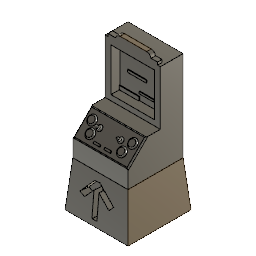
DiegoCabinet (Autodesk Fusion 360 design; units mm, degrees)
Autodesk Fusion 360 part; units mm, degrees
sketch "Sketch1" plane through (0, 0, 0) normal (0, 0, 1) x (1, 0, 0)
  line L0 (0, 50) -> (70, 50)
  line L1 (70, 50) -> (70, -20)
  line L2 (70, -20) -> (0, -20)
  line L3 (0, -20) -> (0, 50)
  constraint horizontal L0
  constraint vertical L1
  constraint horizontal L2
  constraint vertical L3
extrude "Extrude1" add sketch "Sketch1" along normal blind 50 draft -5
sketch "Sketch2" plane through (0, 0, 50) normal (0, 0, 1) x (-1, 0, 0)
  line L0 (-4.3744, -45.6256) -> (-4.3744, 15.6256)
  line L1 (-4.3744, 15.6256) -> (-65.6256, 15.6256)
  line L2 (-65.6256, 15.6256) -> (-65.6256, -45.6256)
  line L3 (-65.6256, -45.6256) -> (-4.3744, -45.6256)
  line L4 (-4.3744, 15.6256) -> (-65.6256, 15.6256)
  line L5 (-65.6256, 15.6256) -> (-65.6256, -45.6256)
  line L6 (-65.6256, -45.6256) -> (-4.3744, -45.6256)
  line L7 (-4.3744, -45.6256) -> (-4.3744, 15.6256)
  constraint horizontal L4
  constraint vertical L5
  constraint horizontal L6
  constraint vertical L7
  constraint coincident L2.end L3.start
  constraint coincident L0.end L1.start
extrude "Extrude2" add sketch "Sketch2" along normal blind 40
chamfer "Chamfer1" distance 20 angle 45 1 edges at (35, -15.6256, 90)
sketch "Sketch3" plane through (0, 0, 90) normal (0, 0, 1) x (-1, 0, 0)
  line L0 (-4.3744, -4.3744) -> (-65.6256, -4.3744)
  line L1 (-65.6256, -4.3744) -> (-65.6256, -45.6256)
  line L2 (-65.6256, -45.6256) -> (-4.3744, -45.6256)
  line L3 (-4.3744, -45.6256) -> (-4.3744, -4.3744)
  line L4 (-65.6256, -20.1653) -> (-4.3744, -20.1653)
  line L5 (-4.3744, -20.1653) -> (-4.3744, -45.6256)
  line L6 (-4.3744, -45.6256) -> (-65.6256, -45.6256)
  line L7 (-65.6256, -45.6256) -> (-65.6256, -20.1653)
  constraint horizontal L4
  constraint vertical L5
  constraint horizontal L6
  constraint vertical L7
  constraint coincident L2.end L3.start
  constraint coincident L1 L4.start
extrude "Extrude3" add sketch "Sketch3" along normal blind 60 contours L1 L2 L3 L4 L5 L6 L7
sketch "Sketch4" plane through (0, -42.8128, 42.8128) normal (0, -0.707107, 0.707107) x (1, 0, 0)
  line L0 (65.6256, 38.4485) -> (65.6256, 66.7328)
  line L1 (65.6256, 66.7328) -> (4.3744, 66.7328)
  line L2 (4.3744, 66.7328) -> (4.3744, 38.4485)
  line L3 (4.3744, 38.4485) -> (65.6256, 38.4485)
  circle A0 centre (52.5, 47.5) radius 3.5355
  circle A1 centre (57.5, 57.5) radius 3.5355
extrude "Extrude4" add sketch "Sketch4" along normal blind 1.5 contours A0 | A1
sketch "Sketch5" plane through (0, -42.8128, 42.8128) normal (0, -0.707107, 0.707107) x (1, 0, 0)
  circle A0 centre (52.5, 47.5) radius 3.5355
  circle A1 centre (57.5, 57.5) radius 3.5355
  line L0 (65.6256, 38.4485) -> (65.6256, 66.7328)
  line L1 (65.6256, 66.7328) -> (4.3744, 66.7328)
  line L2 (4.3744, 66.7328) -> (4.3744, 38.4485)
  line L3 (4.3744, 38.4485) -> (65.6256, 38.4485)
  circle A2 centre (46, 55) radius 1.4142
extrude "Extrude5" add sketch "Sketch5" along normal blind 6 contours A2
fillet "Fillet1" radius 1 1 edges at (44.6815, -8.5262, 85.5847)
sketch "Sketch6" plane through (0, -42.8128, 42.8128) normal (0, -0.707107, 0.707107) x (1, 0, 0)
  circle A0 centre (46, 55) radius 1.4142
  circle A1 centre (52.5, 47.5) radius 3.5355
  circle A2 centre (57.5, 57.5) radius 3.5355
  line L0 (65.6256, 38.4485) -> (65.6256, 66.7328)
  line L1 (65.6256, 66.7328) -> (4.3744, 66.7328)
  line L2 (4.3744, 66.7328) -> (4.3744, 38.4485)
  line L3 (4.3744, 38.4485) -> (65.6256, 38.4485)
  circle A3 centre (17.5, 47.5) radius 3.5355
  circle A4 centre (12.5, 57.5) radius 3.5355
extrude "Extrude6" add sketch "Sketch6" along normal blind 1.5 contours A3 | A4
sketch "Sketch7" plane through (0, -42.8128, 42.8128) normal (0, -0.707107, 0.707107) x (1, 0, 0)
  circle A0 centre (17.5, 47.5) radius 3.5355
  circle A1 centre (12.5, 57.5) radius 3.5355
  circle A2 centre (46, 55) radius 1.4142
  circle A3 centre (52.5, 47.5) radius 3.5355
  circle A4 centre (57.5, 57.5) radius 3.5355
  line L0 (65.6256, 38.4485) -> (65.6256, 66.7328)
  line L1 (65.6256, 66.7328) -> (4.3744, 66.7328)
  line L2 (4.3744, 66.7328) -> (4.3744, 38.4485)
  line L3 (4.3744, 38.4485) -> (65.6256, 38.4485)
  circle A5 centre (22.5, 55) radius 1.5
extrude "Extrude7" add sketch "Sketch7" along normal blind 6 contours A5
fillet "Fillet2" radius 1.5 1 edges at (21.1015, -8.5481, 85.5627)
fillet "Fillet3" radius 1.5 3 faces at (47.165, -7.1419, 85.9531) (47.3705, -6.5257, 83.8139) (46.1219, -8.0981, 86.0127)
fillet "Fillet4" radius 1.5 2 faces at (21.7564, -6.3316, 85.9348) (23.9981, -5.0354, 82.7114)
fillet "Fillet5" radius 1.414 8 faces at (47.165, -7.1419, 85.9531) (46.9358, -6.5573, 82.8395) (48.1777, -2.631, 82.997) (38.4505, 2.2787, 87.9042) (24.999, -2.8433, 82.7847) (23.9981, -5.6368, 83.5243) (21.7564, -6.3316, 85.9348) (46.1219, -8.0981, 86.0127)
sketch "Sketch8" plane through (0, -42.8128, 42.8128) normal (0, -0.707107, 0.707107) x (1, 0, 0)
  circle A0 centre (57.5, 57.5) radius 4.9495
  circle A1 centre (12.5, 57.5) radius 4.9495
  circle A2 centre (22.5, 55) radius 3
  circle A3 centre (46, 55) radius 2.9142
  circle A4 centre (17.5, 47.5) radius 4.9495
  circle A5 centre (52.5, 47.5) radius 4.9495
  line L0 (64.2116, 66.1471) -> (5.7884, 66.1471)
  line L1 (5.7884, 66.1471) -> (5.7884, 39.0342)
  line L2 (5.7884, 39.0342) -> (64.2116, 39.0342)
  line L3 (64.2116, 39.0342) -> (64.2116, 66.1471)
  line L4 (25, 44) -> (32, 44)
  line L5 (32, 44) -> (32, 42)
  line L6 (32, 42) -> (25, 42)
  line L7 (25, 42) -> (25, 44)
  line L8 (37, 44) -> (44, 44)
  line L9 (44, 44) -> (44, 42)
  line L10 (44, 42) -> (37, 42)
  line L11 (37, 42) -> (37, 44)
  constraint horizontal L4
  constraint vertical L5
  constraint horizontal L6
  constraint vertical L7
  constraint horizontal L8
  constraint vertical L9
  constraint horizontal L10
  constraint vertical L11
extrude "Extrude8" add sketch "Sketch8" along normal blind 1 contours L4 L5 L6 L7 | L8 L9 L10 L11
sketch "Sketch9" plane through (0, 20.1653, 0) normal (0, -1, 0) x (1, 0, 0)
  line L0 (4.3744, 90) -> (65.6256, 90)
  line L1 (65.6256, 90) -> (65.6256, 150)
  line L2 (65.6256, 150) -> (4.3744, 150)
  line L3 (4.3744, 150) -> (4.3744, 90)
  line L4 (10.9653, 143.6315) -> (59.1907, 143.6315)
  line L5 (59.1907, 143.6315) -> (59.1907, 95.948)
  line L6 (59.1907, 95.948) -> (10.9653, 95.948)
  line L7 (10.9653, 95.948) -> (10.9653, 143.6315)
  constraint horizontal L4
  constraint vertical L5
  constraint horizontal L6
  constraint vertical L7
extrude "Extrude9" cut sketch "Sketch9" against normal blind 10 contours L4 L5 L6 L7
sketch "Sketch10" plane through (0, 30.1653, 0) normal (0, -1, 0) x (1, 0, 0)
  line L0 (10.9653, 95.948) -> (59.1907, 95.948)
  line L1 (59.1907, 95.948) -> (59.1907, 143.6315)
  line L2 (59.1907, 143.6315) -> (10.9653, 143.6315)
  line L3 (10.9653, 143.6315) -> (10.9653, 95.948)
  line L4 (49.395, 103.1903) -> (32.8683, 103.1903)
  line L5 (32.8683, 103.1903) -> (32.8683, 105.3578)
  line L6 (32.8683, 105.3578) -> (49.395, 105.3578)
  line L7 (49.395, 105.3578) -> (49.395, 103.1903)
  line L8 (10.9653, 100.2101) -> (32.8683, 100.2101)
  line L9 (32.8683, 100.2101) -> (32.8683, 95.948)
  line L10 (32.8683, 95.948) -> (10.9653, 95.948)
  line L11 (10.9653, 95.948) -> (10.9653, 100.2101)
  line L12 (51.8334, 114.0275) -> (59.1907, 114.0275)
  line L13 (59.1907, 114.0275) -> (59.1907, 109.6927)
  line L14 (59.1907, 109.6927) -> (51.8334, 109.6927)
  line L15 (51.8334, 109.6927) -> (51.8334, 114.0275)
  line L16 (20, 120) -> (40.9962, 120)
  line L17 (40.9962, 120) -> (40.9962, 117.2787)
  line L18 (40.9962, 117.2787) -> (20, 117.2787)
  line L19 (20, 117.2787) -> (20, 120)
  constraint horizontal L4
  constraint vertical L5
  constraint horizontal L6
  constraint vertical L7
  constraint horizontal L8
  constraint vertical L9
  constraint horizontal L10
  constraint vertical L11
  constraint coincident L0 L9.end
  constraint coincident L3 L8.start
  constraint horizontal L12
  constraint vertical L13
  constraint horizontal L14
  constraint vertical L15
  constraint coincident L1 L13.end
  constraint horizontal L16
  constraint vertical L17
  constraint horizontal L18
  constraint vertical L19
extrude "Extrude10" add sketch "Sketch10" along normal blind 0.8 contours L0 L3 L8 L9 L10 L11 | L1 L12 L13 L14 L15 | L4 L5 L6 L7 | L16 L17 L18 L19
sketch "Sketch11" plane through (0, 0, 150) normal (0, 0, 1) x (-1, 0, 0)
  line L0 (-65.6256, -45.6256) -> (-4.3744, -45.6256)
  line L1 (-4.3744, -45.6256) -> (-4.3744, -20.1653)
  line L2 (-4.3744, -20.1653) -> (-65.6256, -20.1653)
  line L3 (-65.6256, -20.1653) -> (-65.6256, -45.6256)
  line L4 (-7.7964, -25.1653) -> (-62.5883, -25.1653)
  line L5 (-62.5883, -25.1653) -> (-62.5883, -20.1653)
  line L6 (-62.5883, -20.1653) -> (-7.7964, -20.1653)
  line L7 (-7.7964, -20.1653) -> (-7.7964, -25.1653)
  constraint horizontal L4
  constraint vertical L5
  constraint horizontal L6
  constraint vertical L7
  constraint coincident L2 L5.end
extrude "Extrude11" add sketch "Sketch11" along normal blind 3 contours L2 L4 L5 L6 L7
sketch "Sketch12" plane through (0, 0, 153) normal (0, 0, 1) x (-1, 0, 0)
  line L0 (-7.7964, -20.1653) -> (-62.5883, -20.1653)
  line L1 (-62.5883, -20.1653) -> (-62.5883, -25.1653)
  line L2 (-62.5883, -25.1653) -> (-7.7964, -25.1653)
  line L3 (-7.7964, -25.1653) -> (-7.7964, -20.1653)
  line L4 (-16.1152, -25.1653) -> (-55.3218, -25.1653)
  line L5 (-55.3218, -25.1653) -> (-55.3218, -20.1653)
  line L6 (-55.3218, -20.1653) -> (-16.1152, -20.1653)
  line L7 (-16.1152, -20.1653) -> (-16.1152, -25.1653)
  constraint horizontal L4
  constraint vertical L5
  constraint horizontal L6
  constraint vertical L7
  constraint coincident L0 L5.end
  constraint coincident L2 L4.start
extrude "Extrude12" add sketch "Sketch12" along normal blind 4 contours L0 L2 L4 L5 L6 L7
fillet "Fillet6" radius 5 1 edges at (16.1152, 22.6653, 157)
fillet "Fillet7" radius 5 1 edges at (55.3218, 22.6653, 157)
sketch "Sketch13" plane through (0, 0, 157) normal (0, 0, 1) x (-1, 0, 0)
  line L0 (-50.4228, -20.1653) -> (-50.4228, -25.1653)
  line L1 (-50.4228, -25.1653) -> (-21.0141, -25.1653)
  line L2 (-21.0141, -25.1653) -> (-21.0141, -20.1653)
  line L3 (-21.0141, -20.1653) -> (-50.4228, -20.1653)
sketch "Sketch14" plane through (0, -19.8481, 1.7365) normal (0, -0.996195, 0.087156) x (1, 0, 0)
  line L0 (65.6256, 48.4479) -> (4.3744, 48.4479)
  line L1 (4.3744, 48.4479) -> (0, -1.7431)
  line L2 (0, -1.7431) -> (70, -1.7431)
  line L3 (70, -1.7431) -> (65.6256, 48.4479)
  line L4 (29.5075, 4.3578) -> (35, 4.3578)
  line L5 (35, 4.3578) -> (35, 30.6648)
  line L6 (35, 30.6648) -> (29.5075, 30.6648)
  line L7 (29.5075, 30.6648) -> (29.5075, 4.3578)
  line L8 (0, 4.3578) -> (70, 4.3578)
  constraint horizontal L4
  constraint vertical L5
  constraint horizontal L6
  constraint vertical L7
  constraint coincident L4.start L8
extrude "Extrude13" cut sketch "Sketch14" against normal blind 10 contours L4 L5 L6 L7 L8
sketch "Sketch15" plane through (0, -19.8481, 1.7365) normal (0, -0.996195, 0.087156) x (1, 0, 0)
  line L0 (35, 4.3578) -> (29.5075, 4.3578)
  line L1 (29.5075, 4.3578) -> (29.5075, 30.6648)
  line L2 (29.5075, 30.6648) -> (35, 30.6648)
  line L3 (35, 30.6648) -> (35, 4.3578)
  line L4 (65.6256, 48.4479) -> (4.3744, 48.4479)
  line L5 (4.3744, 48.4479) -> (0, -1.7431)
  line L6 (0, -1.7431) -> (70, -1.7431)
  line L7 (70, -1.7431) -> (65.6256, 48.4479)
  line L8 (20, 20) -> (29.5075, 30.6648)
  line L9 (35, 30.6648) -> (46.963, 20)
  line L10 (46.963, 20) -> (51.7168, 25.3324)
  line L11 (51.7168, 25.3324) -> (35, 40.2352)
  line L12 (35, 40.2352) -> (29.5075, 39.4042)
  line L13 (29.5075, 39.4042) -> (14.5859, 22.6662)
  line L14 (14.5859, 22.6662) -> (20, 20)
  constraint coincident L1.end L2.start
  constraint coincident L2.end L3.start
  constraint perpendicular L8 L9
  constraint perpendicular L9 L10
  constraint perpendicular L10 L11
  constraint perpendicular L9 L13
extrude "Extrude14" cut sketch "Sketch15" against normal blind 10 contours L2 L8 L9 L10 L11 L12 L13 L14
sketch "Sketch16" plane through (69.4683, 0, 6.0777) normal (0.996195, 0, 0.087156) x (0, 1, 0)
  line L0 (45.6256, 44.0901) -> (-15.6256, 44.0901)
  line L1 (-15.6256, 44.0901) -> (-20, -6.1009)
  line L2 (-20, -6.1009) -> (50, -6.1009)
  line L3 (50, -6.1009) -> (45.6256, 44.0901)
